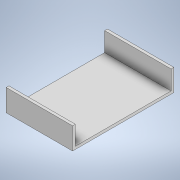
# Autodesk Inventor part: Caja2
Saved by Autodesk Inventor 2021 (Build 250183000, 183)
## iProperties
Created: 2021-02-22
Part Number: Caja2
Material: Generic
Document SubType Name: Modeling
Designer: deuts
Density: 1 g/cm^3
Appearance: Default
Author: deuts
Autodesk Inventor part; units mm, degrees
ref_plane "YZ Plane" through (0, 0, 0) normal (1, 0, 0) x (0, 1, 0)
ref_plane "XZ Plane" through (0, 0, 0) normal (0, 1, 0) x (-1, 0, 0)
ref_plane "XY Plane" through (0, 0, 0) normal (0, 0, 1) x (1, 0, 0)
sketch "Sketch1" plane through (0, 0, 0) normal (0, 1, 0) x (-1, 0, 0)
  line L0 (-60, 91.5) -> (60, 91.5)
  line L1 (60, 91.5) -> (60, -91.5)
  line L2 (60, -91.5) -> (-60, -91.5)
  line L3 (-60, -91.5) -> (-60, 91.5)
  line L4 (-60, 91.5) -> (60, -91.5) construction
  line L5 (60, 91.5) -> (-60, -91.5) construction
  point P0 (0, 0)
  dimension "d0" = 120
  dimension "d1" = 183
  constraints: 12 end point, 2 midpoint, 2 parallel, 1 horizontal, 1 perpendicular
  measures "d0" distance of L1.end L2.end
  measures "d1" distance of L0.end L1.end
extrude "Extrusion1" add sketch "Sketch1" along normal blind 5
sketch "Sketch2" plane through (0, 5, 0) normal (0, 1, 0) x (1, 0, 0)
  line L0 (-60, 91.5) -> (-60, -91.5) projected
  line L1 (60, -91.5) -> (60, 91.5) projected
  line L2 (-60, -91.5) -> (60, -91.5)
  line L3 (60, -91.5) -> (60, -86.5)
  line L4 (60, -86.5) -> (-60, -86.5)
  line L5 (-60, -86.5) -> (-60, -91.5)
  point P0 (0, 0)
  dimension "d4" = 5
  constraints: 8 end point, 2 parallel, 1 horizontal, 1 perpendicular, 1 point on line
  measures "d4" distance of L3.end L2.end
extrude "Extrusion2" add sketch "Sketch2" along normal blind 34.5
sketch "Sketch3" plane through (0, 5, 0) normal (0, 1, 0) x (1, 0, 0)
  line L0 (60, 91.5) -> (-60, 91.5) projected
  line L1 (60, -91.5) -> (60, 91.5) projected
  line L2 (-60, 91.5) -> (60, 91.5)
  line L3 (60, 91.5) -> (60, 86.5)
  line L4 (60, 86.5) -> (-60, 86.5)
  line L5 (-60, 86.5) -> (-60, 91.5)
  point P0 (0, 0)
  dimension "d7" = 5
  constraints: 8 end point, 2 parallel, 1 horizontal, 1 perpendicular, 1 point on line
  measures "d7" distance of L2.end L3.end
extrude "Extrusion3" add sketch "Sketch3" along normal blind 34.5
body "Solid1"
